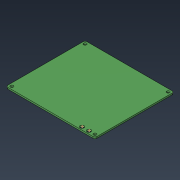
# Autodesk Inventor part: Powerboard
Saved by Autodesk Inventor 2022.1 (Build 261234020, 234B)
## iProperties
Part Number: Powerboard
Material: Phenolharz
Document SubType Name: Modeling
Designer: rYan
Mass: 15.7721 g
Surface Area: 149.254 cm^2
Volume: 11.4291 cm^3
Density: 1.38 g/cm^3
Appearance: Glatt - waldgrün
Categories: <MemberInstance><Categories><Category DisplayName="" Mnemonic="CABLEANDHARNESS" InternalName="e4a7e005-5e42-4d16-b293-125e7f0d0512"><Category DisplayName="" Mnemonic="CONNECTORS" InternalName="6f634eba-a678-4820-a31d-2c2d5ee6728e"><CategoryParameter DisplayName="" Mnemonic="REFDES" InternalName="c3740e8c-60ab-4d5d-8584-52b73222f2f0"/><Category DisplayName="" Mnemonic="DISCRETEWIRE" InternalName="9a3407de-09b2-4cdb-8c40-9708d5144a28"/></Category></Category></Categories><FamilyTemplate><FamilyTemplateParameters></FamilyTemplateParameters></FamilyTemplate><CategoryParameterMap><ParamToTemplateMap><ParamToTemplate CategoryParameter="//CategoryParameter[@InternalName='c3740e8c-60ab-4d5d-8584-52b73222f2f0']" ConstantValue=""/></ParamToTemplateMap></CategoryParameterMap></MemberInstance>
Author: rYan
Autodesk Inventor part; units mm, degrees
ref_plane "YZ Plane" through (0, 0, 0) normal (1, 0, 0) x (0, 1, 0)
ref_plane "XZ Plane" through (0, 0, 0) normal (0, 1, 0) x (-1, 0, 0)
ref_plane "XY Plane" through (0, 0, 0) normal (0, 0, 1) x (1, 0, 0)
sketch "Skizze1" plane through (0, 0, 0) normal (0, 0, 1) x (1, 0, 0)
  line L0 (-45, -37) -> (45, -37)
  line L1 (45, -37) -> (45, 43)
  line L2 (45, 43) -> (-45, 43)
  line L3 (-45, 43) -> (-45, -37)
  line L4 (0, 59) -> (0, -53) projected
  point P0 (0, 0)
  dimension "d0" = 90
  dimension "d2" = 37
  dimension "d14" = 80
  constraints: 8 end point, 2 parallel, 1 horizontal, 1 perpendicular, 1 other
  measures "d0" distance of L2.end L1.end
  measures "d2" distance from line of point (0, 0) L0
  measures "d14" distance of L2.end L0.start
extrude "Extrusion1" add sketch "Skizze1" along normal blind 1.6
sketch "Skizze2" plane through (0, 0, 1.6) normal (0, 0, 1) x (1, 0, 0)
  line L0 (-45, -37) -> (45, -37) projected
  line L1 (45, -37) -> (45, 43) projected
  line L2 (45, 43) -> (-45, 43) projected
  line L3 (-45, 43) -> (-45, -37) projected
  line L4 (-42, -34) -> (42, -34)
  line L5 (42, -34) -> (42, 40)
  line L6 (42, 40) -> (-42, 40)
  line L7 (-42, 40) -> (-42, -34)
  line L8 (0, 59) -> (0, -53) projected
  point P0 (0, 0)
  point P1 (42, -34)
  dimension "d5" = 3
  constraints: 8 end point, 2 coincident, 1 point on line, 1 symmetric about line, 3 other
  measures "d5" distance between parallel lines of L3 L7
hole "Montage" at (-42, 40, 1.6) at (42, 40, 1.6) at (42, -34, 1.6) at (-42, -34, 1.6) direction (0, 0, -1) diameter 3 end through all
sketch "Skizze3" plane through (0, 0, 1.6) normal (0, 0, 1) x (1, 0, 0)
  line L0 (29, -34) -> (36, -34) construction
  circle A0 centre (42, 40) radius 1.5 projected
  circle A1 centre (-42, 40) radius 1.5 projected
  circle A2 centre (42, -34) radius 1.5 projected
  line L1 (-45, -37) -> (45, -37) projected
  line L2 (45, -37) -> (45, 43) projected
  line L3 (45, 43) -> (-45, 43) projected
  line L4 (-45, 43) -> (-45, -37) projected
  point P0 (0, 0)
  dimension "d27" = 7
  dimension "d29" = 3
  dimension "d30" = 9
  constraints: 2 end point, 1 horizontal
  measures "d27" distance of L0.start L0.end
  measures "d29" distance between parallel lines of L1 L0
  measures "d30" distance from line of L2 L0.end
hole "Akku" at (36, -34, 1.6) at (29, -34, 1.6) direction (0, 0, -1) diameter 4 end through all
sketch "Skizze4" plane through (0, 0, 1.6) normal (0, 0, 1) x (1, 0, 0)
  circle A0 centre (29, -34) radius 2 projected
sketch "Skizze5" plane through (0, 0, 1.6) normal (0, 0, 1) x (1, 0, 0)
  circle A0 centre (36, -34) radius 2 projected
fillet "Rundung3" radius 2 4 edges at (45, -37, 0.8) (45, 43, 0.8) (-45, 43, 0.8) (-45, -37, 0.8)
